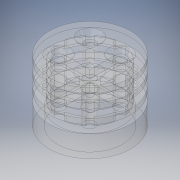
# Autodesk Inventor part: Felga
Saved by Autodesk Inventor 2019 (Build 230136000, 136)
## iProperties
Created: 2021-11-20
Part Number: Felga
Material: Tworzywo sztuczne PMMA
Document SubType Name: Modeling
Designer: Michał
Density: 1.188 g/cm^3
Appearance: Poliwęglan — przezroczysty
Author: Michał
Autodesk Inventor part; units mm, degrees
ref_plane "YZ Plane" through (0, 0, 0) normal (1, 0, 0) x (0, 1, 0)
sketch "Szkic1" plane through (0, 0, 0) normal (0, 1, 0) x (-1, 0, 0)
  circle A0 centre (0, 0) radius 12.5
  circle A1 centre (0, 0) radius 10
  dimension "d0" = 20
  dimension "d2" = 25
  constraints: 2 centre point, 2 coincident
  measures "d0" diameter of A1
  measures "d2" diameter of A0
extrude "Wyciągnięcie proste1" add sketch "Szkic1" along normal blind 5
ref_plane "Płaszczyzna konstrukcyjna1" through (0, -12, 0) normal (0, 0, -1) x (-1, 0, 0)
sketch "Szkic5" plane through (0, -12, 0) normal (0, 0, -1) x (-1, 0, 0)
  line L0 (12.5, 17) -> (-12.5, 17) projected
  line L1 (0, 17) -> (-12.5, 17)
  line L2 (-12.5, 17) -> (-12.5, 18.625)
  line L3 (-12.5, 18.625) -> (0, 18.625)
  line L4 (0, 18.625) -> (0, 17)
  line L5 (0, 18.625) -> (-9.5, 18.625)
  line L6 (-9.5, 18.625) -> (-9.5, 21.125)
  line L7 (-9.5, 21.125) -> (0, 21.125)
  line L8 (0, 21.125) -> (0, 18.625)
  line L9 (0, 21.125) -> (-12.5, 21.125)
  line L10 (-12.5, 21.125) -> (-12.5, 22.75)
  line L11 (-12.5, 22.75) -> (0, 22.75)
  line L12 (0, 22.75) -> (0, 21.125)
  line L13 (0, 22.75) -> (-9.5, 22.75)
  line L14 (-9.5, 22.75) -> (-9.5, 25.25)
  line L15 (-9.5, 25.25) -> (0, 25.25)
  line L16 (0, 25.25) -> (0, 22.75)
  line L17 (0, 25.25) -> (-12.5, 25.25)
  line L18 (-12.5, 25.25) -> (-12.5, 26.875)
  line L19 (-12.5, 26.875) -> (0, 26.875)
  line L20 (0, 26.875) -> (0, 25.25)
  line L21 (0, 26.875) -> (-9.5, 26.875)
  line L22 (-9.5, 26.875) -> (-9.5, 29.375)
  line L23 (-9.5, 29.375) -> (0, 29.375)
  line L24 (0, 29.375) -> (0, 26.875)
  line L25 (0, 29.375) -> (-12.5, 29.375)
  line L26 (-12.5, 29.375) -> (-12.5, 31)
  line L27 (-12.5, 31) -> (0, 31)
  line L28 (0, 31) -> (0, 29.375)
  line L29 (-12.5, 12) -> (-12.5, 17) construction
  line L30 (-12.5, 12) -> (-12.5, 17) construction
  line L31 (-12.5, 12) -> (12.5, 12) construction
  point P0 (0, 12)
  dimension "d13" = 2.5
  dimension "d17" = 19
  dimension "d18" = 3
  constraints: 58 end point, 15 equal length, 7 horizontal, 7 perpendicular, 6 point on line, 5 collinear, 1 midpoint
  measures "d13" distance of L5.end L6.end
  measures "d17" distance between parallel lines of L27 L31
  measures "d18" distance between parallel lines of L26 L22
revolve "Obrót1" add sketch "Szkic5" angle 360 about axis through (0, 10.75, 0) along (0, -1, 0)
sketch "Szkic7" plane through (0, 17.375, 0) normal (0, -1, 0) x (1, 0, 0)
  circle A0 centre (0, 0) radius 9.5 projected
  circle A1 centre (0, 9.5) radius 1.65
  circle A2 centre (0, 0) radius 10 projected
  circle A3 centre (0, 0) radius 9.5 projected
  circle A4 centre (-9.5, 0) radius 1.65
  circle A5 centre (0, -9.5) radius 1.65
  circle A6 centre (9.5, 0) radius 1.65
  circle A7 centre (6.7175, -6.7175) radius 0.9
  circle A8 centre (6.7175, 6.7175) radius 0.9
  circle A9 centre (-6.7175, 6.7175) radius 0.9
  circle A10 centre (-6.7175, -6.7175) radius 0.9
  line L0 (6.7175, 6.7175) -> (0, 0) construction
  line L1 (0, 0) -> (-6.7175, 6.7175) construction
  circle A11 centre (0, 0) radius 12.5 construction
  line L2 (0, 0) -> (-6.7175, -6.7175) construction
  line L3 (0, 0) -> (6.7175, -6.7175) construction
  line L4 (17.5, 0) -> (-17.5, 0) construction
  dimension "d23" = 45
  dimension "d24" = 45
  dimension "d25" = 3.3
  dimension "d47" = 1.8
  constraints: 8 centre point, 8 end point, 8 point on circle, 6 equal radius, 2 collinear
  measures "d23" angle of L4 L1
  measures "d24" angle of L0 L4
  measures "d25" diameter of A1
  measures "d47" diameter of A9
extrude "Wyciągnięcie proste6" cut sketch "Szkic7" along normal up to surface (10.75 mm away) contours A0 A6 | A0 A6 A2 | A8 A0 | A0 A8 A2 | A6 A2 | A7 A2 A0 | A0 A7 | A2 A8 | A7 A2 | A1 A0 | A0 A1 A2 | A5 A2 A0 | A0 A5 | A2 A1 | A5 A2 | A9 A0 | A0 A9 A2 | A10 A2 A0 | A0 A10 | A2 A9 | A10 A2 | A4 A0 | A0 A4 A2 | A2 A4
sketch "Szkic8" plane through (0, -12, 0) normal (0, 0, -1) x (-1, 0, 0)
  line L0 (6.0517, 25.25) -> (1.6438, 25.25) projected
  line L1 (-1.6438, 25.25) -> (-1.6438, 22.75) projected
  line L2 (1.6438, 25.25) -> (-1.6438, 25.25)
  line L3 (-1.6438, 25.25) -> (-1.6438, 22.75)
  line L4 (-1.6438, 22.75) -> (1.6438, 22.75)
  line L5 (1.6438, 22.75) -> (1.6438, 25.25)
  point P0 (0, 12)
  point P1 (1.65, 22.75)
  constraints: 8 end point, 2 parallel, 1 horizontal, 1 perpendicular
extrude "Wyciągnięcie proste7" cut sketch "Szkic8" along normal through all both and the other way through all
sketch "Szkic9" plane through (0, 5, 0) normal (0, -1, 0) x (1, 0, 0)
  line L0 (0, 0) -> (-3.4352, 0)
  line L1 (-3.4352, 0) -> (-3.4352, -2.2657)
  line L2 (-3.4352, -2.2657) -> (0, -2.2657)
  line L3 (0, -2.2657) -> (0, 0)
  dimension "d30" = 3.4352
  dimension "d31" = 2.2658
  constraints: 8 end point, 2 parallel, 1 horizontal, 1 perpendicular
  measures "d30" distance of L1.end L2.end
  measures "d31" distance of L0.end L1.end
extrude "Wyciągnięcie proste8" add sketch "Szkic9" along normal blind 15
ref_plane "Płaszczyzna konstrukcyjna2" through (0, -10, -2.2657) normal (1, 0, 0) x (0, 0, -1)
sketch "Szkic10" plane through (0, -10, 0) normal (0, -1, 0) x (1, 0, 0)
  line L0 (0, 0) -> (-3.4352, 0) projected
  line L1 (-3.4352, -2.2657) -> (0, -2.2657) projected
  line L2 (0, 0) -> (-3.4352, 0)
  line L3 (-3.4352, 0) -> (-3.4352, -2.2657)
  line L4 (-3.4352, -2.2657) -> (0, -2.2657)
  line L5 (0, -2.2657) -> (0, 0)
  constraints: 8 end point, 2 parallel, 1 horizontal, 1 perpendicular
extrude "Wyciągnięcie proste9" cut sketch "Szkic10" against normal up to surface (15 mm away)
sketch "Szkic11" plane through (0, -10, -2.2657) normal (1, 0, 0) x (0, 0, -1)
  line L0 (-3.9095, 20.75) -> (-3.9095, 23.25) projected
  line L1 (-0.622, 20.75) -> (-0.622, 23.25) projected
  line L2 (-3.9095, 20.75) -> (-0.622, 20.75)
  line L3 (-0.622, 20.75) -> (-0.622, 23.25)
  line L4 (-0.622, 23.25) -> (-3.9095, 23.25)
  line L5 (-3.9095, 23.25) -> (-3.9095, 20.75)
  point P0 (-2.2657, 10)
  constraints: 8 end point, 2 parallel, 1 horizontal, 1 perpendicular
extrude "Wyciągnięcie proste10" cut sketch "Szkic11" along normal through all both and the other way through all
sketch "Szkic12" plane through (0, 19, 0) normal (0, 1, 0) x (1, 0, 0)
  line L0 (0, 0) -> (4.6374, 4.6374) construction
  line L1 (0, 0) -> (6.5583, 0) construction
  line L2 (0, 0) -> (-4.6374, 4.6374) construction
  line L3 (0, 0) -> (-4.8503, -4.8503) construction
  line L4 (0, 0) -> (4.8503, -4.8503) construction
  point P0 (-4.6374, 4.6374)
  point P1 (4.6328, -4.7775)
  dimension "d39" = 6.5583
  constraints: 10 end point, 4 coincident, 3 equal length, 2 collinear, 1 perpendicular, 1 point on line
  measures "d39" distance of L1.end L0.start
hole "Otwór1" at (4.6374, 19, -4.6374) at (-4.6374, 19, -4.6374) at (-4.8503, 19, 4.8503) at (4.6328, 19, 4.7775) direction (0, -1, 0) diameter 3.4 end through all countersink diameter 6.9 countersink angle 89.954 clearance for "Śruba ze łbem stożkowym ISO 2009/7046" size "M3" standard "ISO"
sketch "Szkic13" plane through (0, 5, 0) normal (0, -1, 0) x (1, 0, 0)
  circle A0 centre (0, 0) radius 2
  dimension "d48" = 4
  constraints: 1 centre point, 1 coincident
  measures "d48" diameter of A0
extrude "Wyciągnięcie proste11" cut sketch "Szkic13" against normal blind 5
